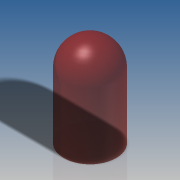
# Autodesk Inventor part: 11177-TransRed
Saved by Autodesk Inventor 2016 SP2 (Build 200236200, 236)
## iProperties
Created: 2015-08-19
Part Number: 11177-TransRed
Material: Polycarbonate
Document SubType Name: Modeling
Designer: D. Kohfeld
Mass: 0.0488983 g
Surface Area: 0.643398 cm^2
Volume: 0.0407486 cm^3
Density: 1.2 g/cm^3
Appearance: TransRed
Author: D. Kohfeld
Autodesk Inventor part; units mm, degrees
ref_plane "YZ Plane" through (0, 0, 0) normal (1, 0, 0) x (0, 1, 0)
ref_plane "XZ Plane" through (0, 0, 0) normal (0, 1, 0) x (-1, 0, 0)
ref_plane "XY Plane" through (0, 0, 0) normal (0, 0, 1) x (1, 0, 0)
sketch "Sketch2" plane through (0, 0, 0) normal (0, 0, 1) x (1, 0, 0)
  line L0 (0, -4) -> (0, 1.6)
  arc A0 (1.6, 0) -> (0, 1.6) centre (0, 0) ccw
  line L1 (1.6, 0) -> (1.6, -4)
  line L2 (1.6, -4) -> (0, -4)
  dimension "d0" = 3.2
  dimension "d1" = 5.6
  constraints: 6 end point, 2 point on circle, 2 vertical, 1 centre point, 1 coincident, 1 horizontal, 1 point on line, 1 tangent
  measures "d0" diameter of L1 L0
  measures "d1" distance from line of L0.end L2
revolve "Revolution1" add sketch "Sketch2" angle 360 about axis through (0, -4, 0) along (0, 1, 0)
body "Solid1"
